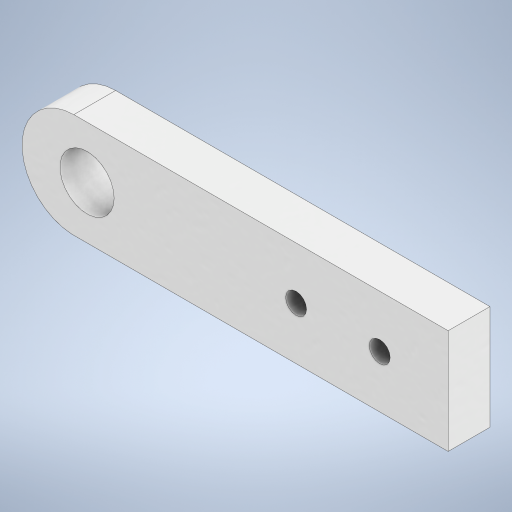
# Autodesk Inventor part: bearing holder (treadmill)
Saved by Autodesk Inventor 2023 (Build 270158000, 158)
## iProperties
Created: 2023-01-12
Part Number: bearing holder (treadmill)
Material: Generic
Document SubType Name: Modeling
Designer: rosam
Density: 1 g/cm^3
Appearance: Default
Autodesk Inventor part; units mm, degrees
ref_plane "YZ Plane" through (0, 0, 0) normal (1, 0, 0) x (0, 1, 0)
ref_plane "XZ Plane" through (0, 0, 0) normal (0, 1, 0) x (-1, 0, 0)
ref_plane "XY Plane" through (0, 0, 0) normal (0, 0, 1) x (1, 0, 0)
sketch "Sketch1" plane through (0, 0, 0) normal (0, 0, 1) x (1, 0, 0)
  circle A0 centre (-138.4817, 178.0572) radius 3.175
  circle A1 centre (-163.8817, 178.0572) radius 3.175
  ellipse E0 centre (-227.3817, 178.0572) end of major axis (-227.3817, 186.291) minor radius 8.1705
  line L0 (-232.0049, 162.186) -> (-232.0049, 162.1895)
  line L1 (-232.0049, 193.9286) -> (-232.0049, 193.9322)
  arc A2 (-231.4064, 193.9395) -> (-232.0049, 162.1895) centre (-231.2487, 178.0559) ccw
  line L2 (-231.4064, 193.9395) -> (-117.7018, 193.9395)
  line L3 (-232.0049, 162.1895) -> (-117.7018, 162.1895)
  line L4 (-117.7018, 193.9395) -> (-117.7018, 162.1895)
  circle A3 centre (-163.8817, 178.0572) radius 3.175
  circle A4 centre (-138.4817, 178.0572) radius 3.175
  circle A5 centre (-227.3817, 178.0572) radius 8.2338
  point P0 (0, 0)
  constraints: 10 end point, 6 centre point, 3 coincident, 2 concentric, 2 horizontal, 2 point on circle, 1 vertical, 3 other
extrude "Extrusion1" add sketch "Sketch1" along normal blind 12.7
body "Solid1"
